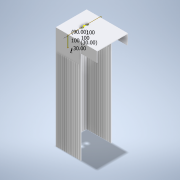
# Autodesk Inventor part: Sensors Holder V2
Saved by Autodesk Inventor 2020 (Build 240168000, 168)
## iProperties
Created: 2020-08-04
Part Number: Sensors Holder V2
Material: Generic
Document SubType Name: Modeling
Designer: Abbas
Density: 1 g/cm^3
Appearance: Default
Author: Abbas
Autodesk Inventor part; units mm, degrees
ref_plane "YZ Plane" through (0, 0, 0) normal (1, 0, 0) x (0, 1, 0)
ref_plane "XZ Plane" through (0, 0, 0) normal (0, 1, 0) x (-1, 0, 0)
ref_plane "XY Plane" through (0, 0, 0) normal (0, 0, 1) x (1, 0, 0)
sketch "Sketch1" plane through (0, 0, 0) normal (0, 1, 0) x (-1, 0, 0)
  line L0 (100, 75) -> (-100, 75)
  line L1 (-100, 75) -> (-100, -75)
  line L2 (-100, -75) -> (100, -75)
  line L3 (100, -75) -> (100, 75)
  line L4 (100, 75) -> (-100, -75) construction
  line L5 (-100, 75) -> (100, -75) construction
  line L6 (-23, 75) -> (-26, 75)
  line L7 (-26, 75) -> (-26, -75)
  line L8 (-26, -75) -> (-23, -75)
  line L9 (-23, -72) -> (-23, 75)
  line L10 (-23, 75) -> (-26, -75) construction
  line L11 (-26, 75) -> (-23, -75) construction
  line L12 (-26, 72) -> (-100, 72)
  line L13 (-100, -72) -> (-26, -72)
  line L14 (-23, -72) -> (-23, -75)
  point P0 (0, 0)
  point P1 (-24.5, 0)
  point P2 (-26, -72)
  point P3 (-26, 72)
  dimension "d11" = 200
  dimension "d12" = 150
  dimension "d18" = 3
  dimension "d19" = 150
  constraints: 30 end point, 5 parallel, 5 point on line, 4 midpoint, 3 horizontal, 2 perpendicular, 1 vertical
  measures "d11" distance of L2.end L1.end
  measures "d12" distance of L1.end L0.end
  measures "d18" distance of L8.end L7.end
  measures "d19" distance of L7.end L6.end
extrude "Extrusion5" add sketch "Sketch1" against normal blind 3 contours L3 L2 L14 L9 L0
extrude "Extrusion6" add sketch "Sketch1" against normal blind 3 contours L7 L13 L1 L12
extrude "Extrusion7" add sketch "Sketch1" against normal blind 50 contours L9 L14 L2 L7 L0 | L7 L12 L1 L0 | L2 L1 L13 L7
sketch "Sketch2" plane through (0, -3, 0) normal (0, -1, 0) x (1, 0, 0)
  line L0 (21, 72) -> (-97, 72)
  line L1 (-97, 72) -> (-97, -72)
  line L2 (-97, -72) -> (21, -72)
  line L3 (21, 72) -> (-97, -72) construction
  line L4 (-97, 72) -> (21, -72) construction
  line L5 (23, 75) -> (-100, 75) projected
  line L6 (-100, -75) -> (23, -75) projected
  line L7 (-100, 75) -> (-100, -75) projected
  line L8 (23, -75) -> (23, 75) projected
  line L9 (21, -75) -> (21, -72)
  line L10 (21, 72) -> (21, 75)
  point P0 (0, 0)
  point P1 (-38, 0)
  dimension "d36" = 3
  dimension "d37" = 3
  dimension "d38" = 3
  constraints: 14 end point, 3 parallel, 2 midpoint, 2 point on line, 1 horizontal, 1 perpendicular
  measures "d36" distance between parallel lines of L5 L0
  measures "d37" distance between parallel lines of L6 L2
  measures "d38" distance between parallel lines of L1 L7
extrude "Extrusion8" add sketch "Sketch2" along normal blind 498 contours L0 L1 L2 L9 L6 L7 L5 L10
sketch "Sketch3" plane through (0, -3, 0) normal (0, -1, 0) x (1, 0, 0)
  circle A0 centre (-37, -12.655) radius 8.2
  circle A1 centre (-37, 12.655) radius 8.2
  line L0 (-43.0434, -5.9922) -> (-47.6499, -5.9922)
  line L1 (-47.6499, -5.9922) -> (-47.6499, 6.0078)
  line L2 (-47.6499, 6.0078) -> (-43.0434, 6.0078)
  line L3 (-43.0434, 6.0078) -> (-43.0434, -5.9922)
  line L4 (-43.0434, -5.9922) -> (-47.6499, 6.0078) construction
  line L5 (-47.6499, -5.9922) -> (-43.0434, 6.0078) construction
  line L6 (-97, -72) -> (-97, 72) projected
  line L7 (-37, 12.655) -> (-37, -12.655)
  point P0 (0, 0)
  point P1 (-45.3467, 0.0078)
  dimension "d42" = 16.4
  dimension "d43" = 16.4
  dimension "d44" = 25.31
  dimension "d45" = 4.6065
  dimension "d46" = 12
  dimension "d47" = 12.6628
  dimension "d48" = 8.3467
  constraints: 14 end point, 2 centre point, 2 midpoint, 2 parallel, 1 horizontal, 1 perpendicular, 1 vertical
  measures "d42" diameter of A0
  measures "d43" diameter of A1
  measures "d44" distance of L7.start L7.end
  measures "d45" distance of L1.end L2.end
  measures "d46" distance of L0.end L1.end
  measures "d47" vertical distance of point (-45.347, 0.008) L7.end
  measures "d48" horizontal distance of L7.end point (-45.347, 0.008)
extrude "Extrusion9" cut sketch "Sketch3" against normal mid plane 20
sketch "Sketch5" plane through (-100, 0, 75) normal (0, 0, 1) x (1, 0, 0)
  line L0 (9.5, -101) -> (12.5, -101)
  line L1 (12.5, -101) -> (12.5, -501)
  line L2 (12.5, -501) -> (9.5, -501)
  line L3 (9.5, -501) -> (9.5, -101)
  line L4 (9.5, -101) -> (12.5, -501) construction
  line L5 (12.5, -101) -> (9.5, -501) construction
  line L6 (121, -501) -> (0, -501) projected
  line L7 (0, 0) -> (0, -501) projected
  line L8 (18.5, -101) -> (21.5, -101)
  line L9 (21.5, -101) -> (21.5, -501)
  line L10 (18.5, -501) -> (18.5, -101)
  line L11 (18.5, -101) -> (21.5, -501) construction
  line L12 (21.5, -101) -> (18.5, -501) construction
  line L13 (21.5, -501) -> (18.5, -501)
  line L14 (27.5, -101) -> (30.5, -101)
  line L15 (30.5, -101) -> (30.5, -501)
  line L16 (27.5, -501) -> (27.5, -101)
  line L17 (27.5, -101) -> (30.5, -501) construction
  line L18 (30.5, -101) -> (27.5, -501) construction
  line L19 (30.5, -501) -> (27.5, -501)
  line L20 (36.5, -101) -> (39.5, -101)
  line L21 (39.5, -101) -> (39.5, -501)
  line L22 (36.5, -501) -> (36.5, -101)
  line L23 (36.5, -101) -> (39.5, -501) construction
  line L24 (39.5, -101) -> (36.5, -501) construction
  line L25 (39.5, -501) -> (36.5, -501)
  line L26 (45.5, -101) -> (48.5, -101)
  line L27 (48.5, -101) -> (48.5, -501)
  line L28 (45.5, -501) -> (45.5, -101)
  line L29 (45.5, -101) -> (48.5, -501) construction
  line L30 (48.5, -101) -> (45.5, -501) construction
  line L31 (48.5, -501) -> (45.5, -501)
  line L32 (54.5, -101) -> (57.5, -101)
  line L33 (57.5, -101) -> (57.5, -501)
  line L34 (54.5, -501) -> (54.5, -101)
  line L35 (54.5, -101) -> (57.5, -501) construction
  line L36 (57.5, -101) -> (54.5, -501) construction
  line L37 (57.5, -501) -> (54.5, -501)
  line L38 (63.5, -101) -> (66.5, -101)
  line L39 (66.5, -101) -> (66.5, -501)
  line L40 (63.5, -501) -> (63.5, -101)
  line L41 (63.5, -101) -> (66.5, -501) construction
  line L42 (66.5, -101) -> (63.5, -501) construction
  line L43 (66.5, -501) -> (63.5, -501)
  line L44 (72.5, -101) -> (75.5, -101)
  line L45 (75.5, -101) -> (75.5, -501)
  line L46 (72.5, -501) -> (72.5, -101)
  line L47 (72.5, -101) -> (75.5, -501) construction
  line L48 (75.5, -101) -> (72.5, -501) construction
  line L49 (75.5, -501) -> (72.5, -501)
  line L50 (81.5, -101) -> (84.5, -101)
  line L51 (84.5, -101) -> (84.5, -501)
  line L52 (81.5, -501) -> (81.5, -101)
  line L53 (81.5, -101) -> (84.5, -501) construction
  line L54 (84.5, -101) -> (81.5, -501) construction
  line L55 (84.5, -501) -> (81.5, -501)
  line L56 (90.5, -101) -> (93.5, -101)
  line L57 (93.5, -101) -> (93.5, -501)
  line L58 (90.5, -501) -> (90.5, -101)
  line L59 (90.5, -101) -> (93.5, -501) construction
  line L60 (93.5, -101) -> (90.5, -501) construction
  line L61 (93.5, -501) -> (90.5, -501)
  line L62 (99.5, -101) -> (102.5, -101)
  line L63 (102.5, -101) -> (102.5, -501)
  line L64 (99.5, -501) -> (99.5, -101)
  line L65 (99.5, -101) -> (102.5, -501) construction
  line L66 (102.5, -101) -> (99.5, -501) construction
  line L67 (102.5, -501) -> (99.5, -501)
  line L68 (108.5, -101) -> (111.5, -101)
  line L69 (111.5, -101) -> (111.5, -501)
  line L70 (108.5, -501) -> (108.5, -101)
  line L71 (108.5, -101) -> (111.5, -501) construction
  line L72 (111.5, -101) -> (108.5, -501) construction
  line L73 (111.5, -501) -> (108.5, -501)
  point P0 (100, 0)
  point P1 (11, -301)
  point P2 (11, -501)
  point P3 (20, -301)
  point P4 (20, -501)
  point P5 (29, -301)
  point P6 (29, -501)
  point P7 (38, -301)
  point P8 (38, -501)
  point P9 (47, -301)
  point P10 (47, -501)
  point P11 (56, -301)
  point P12 (56, -501)
  point P13 (65, -301)
  point P14 (65, -501)
  point P15 (74, -301)
  point P16 (74, -501)
  point P17 (83, -301)
  point P18 (83, -501)
  point P19 (92, -301)
  point P20 (92, -501)
  point P21 (101, -301)
  point P22 (101, -501)
  point P23 (110, -301)
  point P24 (110, -501)
  point P25 (57.5, -501)
  dimension "d63" = 3
  dimension "d64" = 400
  dimension "d65" = 9.5
  dimension "d68" = 9
  constraints: 144 end point, 66 horizontal alignment, 46 parallel, 25 midpoint, 22 collinear, 1 horizontal, 1 perpendicular, 2 other
  measures "d63" distance of L1.end L2.end
  measures "d64" distance of L0.end L1.end
  measures "d65" distance between parallel lines of L7 L3
  measures "d68" distance of L0.start L8.start
extrude "Extrusion10" cut sketch "Sketch5" against normal mid plane 500
sketch "Sketch6" plane through (-100, 0, -75) normal (-1, 0, 0) x (0, 0, 1)
  line L0 (10.5, -101) -> (13.5, -101)
  line L1 (13.5, -101) -> (13.5, -501)
  line L2 (13.5, -501) -> (10.5, -501)
  line L3 (10.5, -501) -> (10.5, -101)
  line L4 (10.5, -101) -> (13.5, -501) construction
  line L5 (13.5, -101) -> (10.5, -501) construction
  line L6 (150, -501) -> (0, -501) projected
  line L7 (0, 0) -> (0, -501) projected
  line L8 (19.5, -101) -> (22.5, -101)
  line L9 (22.5, -101) -> (22.5, -501)
  line L10 (19.5, -501) -> (19.5, -101)
  line L11 (19.5, -101) -> (22.5, -501) construction
  line L12 (22.5, -101) -> (19.5, -501) construction
  line L13 (22.5, -501) -> (19.5, -501)
  line L14 (28.5, -101) -> (31.5, -101)
  line L15 (31.5, -101) -> (31.5, -501)
  line L16 (28.5, -501) -> (28.5, -101)
  line L17 (28.5, -101) -> (31.5, -501) construction
  line L18 (31.5, -101) -> (28.5, -501) construction
  line L19 (31.5, -501) -> (28.5, -501)
  line L20 (37.5, -101) -> (40.5, -101)
  line L21 (40.5, -101) -> (40.5, -501)
  line L22 (37.5, -501) -> (37.5, -101)
  line L23 (37.5, -101) -> (40.5, -501) construction
  line L24 (40.5, -101) -> (37.5, -501) construction
  line L25 (40.5, -501) -> (37.5, -501)
  line L26 (46.5, -101) -> (49.5, -101)
  line L27 (49.5, -101) -> (49.5, -501)
  line L28 (46.5, -501) -> (46.5, -101)
  line L29 (46.5, -101) -> (49.5, -501) construction
  line L30 (49.5, -101) -> (46.5, -501) construction
  line L31 (49.5, -501) -> (46.5, -501)
  line L32 (55.5, -101) -> (58.5, -101)
  line L33 (58.5, -101) -> (58.5, -501)
  line L34 (55.5, -501) -> (55.5, -101)
  line L35 (55.5, -101) -> (58.5, -501) construction
  line L36 (58.5, -101) -> (55.5, -501) construction
  line L37 (58.5, -501) -> (55.5, -501)
  line L38 (64.5, -101) -> (67.5, -101)
  line L39 (67.5, -101) -> (67.5, -501)
  line L40 (64.5, -501) -> (64.5, -101)
  line L41 (64.5, -101) -> (67.5, -501) construction
  line L42 (67.5, -101) -> (64.5, -501) construction
  line L43 (67.5, -501) -> (64.5, -501)
  line L44 (73.5, -101) -> (76.5, -101)
  line L45 (76.5, -101) -> (76.5, -501)
  line L46 (73.5, -501) -> (73.5, -101)
  line L47 (73.5, -101) -> (76.5, -501) construction
  line L48 (76.5, -101) -> (73.5, -501) construction
  line L49 (76.5, -501) -> (73.5, -501)
  line L50 (82.5, -101) -> (85.5, -101)
  line L51 (85.5, -101) -> (85.5, -501)
  line L52 (82.5, -501) -> (82.5, -101)
  line L53 (82.5, -101) -> (85.5, -501) construction
  line L54 (85.5, -101) -> (82.5, -501) construction
  line L55 (85.5, -501) -> (82.5, -501)
  line L56 (91.5, -101) -> (94.5, -101)
  line L57 (94.5, -101) -> (94.5, -501)
  line L58 (91.5, -501) -> (91.5, -101)
  line L59 (91.5, -101) -> (94.5, -501) construction
  line L60 (94.5, -101) -> (91.5, -501) construction
  line L61 (94.5, -501) -> (91.5, -501)
  line L62 (100.5, -101) -> (103.5, -101)
  line L63 (103.5, -101) -> (103.5, -501)
  line L64 (100.5, -501) -> (100.5, -101)
  line L65 (100.5, -101) -> (103.5, -501) construction
  line L66 (103.5, -101) -> (100.5, -501) construction
  line L67 (103.5, -501) -> (100.5, -501)
  line L68 (109.5, -101) -> (112.5, -101)
  line L69 (112.5, -101) -> (112.5, -501)
  line L70 (109.5, -501) -> (109.5, -101)
  line L71 (109.5, -101) -> (112.5, -501) construction
  line L72 (112.5, -101) -> (109.5, -501) construction
  line L73 (112.5, -501) -> (109.5, -501)
  line L74 (118.5, -101) -> (121.5, -101)
  line L75 (121.5, -101) -> (121.5, -501)
  line L76 (118.5, -501) -> (118.5, -101)
  line L77 (118.5, -101) -> (121.5, -501) construction
  line L78 (121.5, -101) -> (118.5, -501) construction
  line L79 (121.5, -501) -> (118.5, -501)
  line L80 (127.5, -101) -> (130.5, -101)
  line L81 (130.5, -101) -> (130.5, -501)
  line L82 (127.5, -501) -> (127.5, -101)
  line L83 (127.5, -101) -> (130.5, -501) construction
  line L84 (130.5, -101) -> (127.5, -501) construction
  line L85 (130.5, -501) -> (127.5, -501)
  line L86 (136.5, -101) -> (139.5, -101)
  line L87 (139.5, -101) -> (139.5, -501)
  line L88 (136.5, -501) -> (136.5, -101)
  line L89 (136.5, -101) -> (139.5, -501) construction
  line L90 (139.5, -101) -> (136.5, -501) construction
  line L91 (139.5, -501) -> (136.5, -501)
  point P0 (75, 0)
  point P1 (12, -301)
  point P2 (12, -501)
  point P3 (21, -301)
  point P4 (21, -501)
  point P5 (30, -301)
  point P6 (30, -501)
  point P7 (39, -301)
  point P8 (39, -501)
  point P9 (48, -301)
  point P10 (48, -501)
  point P11 (57, -301)
  point P12 (57, -501)
  point P13 (66, -301)
  point P14 (66, -501)
  point P15 (75, -301)
  point P16 (75, -501)
  point P17 (84, -301)
  point P18 (84, -501)
  point P19 (93, -301)
  point P20 (93, -501)
  point P21 (102, -301)
  point P22 (102, -501)
  point P23 (111, -301)
  point P24 (111, -501)
  point P25 (120, -301)
  point P26 (120, -501)
  point P27 (129, -301)
  point P28 (129, -501)
  point P29 (138, -301)
  point P30 (138, -501)
  point P31 (31.5, -501)
  point P32 (19.5, -501)
  dimension "d75" = 3
  dimension "d76" = 400
  dimension "d77" = 10.5
  dimension "d80" = 9
  constraints: 180 end point, 84 horizontal alignment, 58 parallel, 31 midpoint, 28 collinear, 1 horizontal, 1 perpendicular, 2 other
  measures "d75" distance of L1.end L2.end
  measures "d76" distance of L0.end L1.end
  measures "d77" distance between parallel lines of L7 L3
  measures "d80" distance of L0.start L8.start
extrude "Extrusion11" cut sketch "Sketch6" along normal mid plane 500
ref_plane "Work Plane1" through (-37, -50, -75) normal (-1, 0, 0) x (0, 0, 1)
sketch "Sketch7" plane through (-37, -50, -75) normal (-1, 0, 0) x (0, 0, 1)
  line L0 (81.0078, 47) -> (69.0078, 47) projected
  line L1 (75.0078, 47) -> (125.0078, -39.6025)
  line L2 (75.0078, 47) -> (175.0078, 47) construction
  line L3 (75.0078, 47) -> (75.0078, -53)
  line L4 (69.0078, 50) -> (81.0078, 50) projected
  line L5 (75.0078, 47) -> (175.0078, 47) construction
  line L6 (75.0078, 47) -> (25.0078, -39.6025)
  line L7 (75.0078, 47) -> (175.0078, 47) construction
  point P0 (75, 50)
  dimension "d89" = 100
  dimension "d91" = 100
  dimension "d93" = 100
  dimension "d94" = 30
  dimension "d95" = 90
  dimension "d96" = 30
  constraints: 12 end point, 3 equal length, 3 horizontal, 1 midpoint, 1 perpendicular
  measures "d89" distance of L1.start L3.end
  measures "d91" distance of L1.start L6.end
  measures "d93" distance of L1.start L1.end
  measures "d94" angle of L3 L6
  measures "d95" angle of L2 L3
  measures "d96" angle of L1 L3
body "Solid2"
